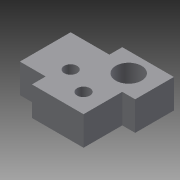
# Autodesk Inventor part: P1-4
Saved by Autodesk Inventor 2014 (Build 180170000, 170)
## iProperties
Created: 2017-02-06
Part Number: P1-4
Material: Generic
Document SubType Name: Modeling
Designer: mschaffel
Density: 1 g/cm^3
Appearance: Default
Author: mschaffel
Autodesk Inventor part; units mm, degrees
ref_plane "YZ Plane" through (0, 0, 0) normal (1, 0, 0) x (0, 1, 0)
ref_plane "XZ Plane" through (0, 0, 0) normal (0, 1, 0) x (-1, 0, 0)
ref_plane "XY Plane" through (0, 0, 0) normal (0, 0, 1) x (1, 0, 0)
sketch "Sketch1" plane through (0, 0, 0) normal (0, 1, 0) x (-1, 0, 0)
  line L0 (0, 0) -> (0, 38.1)
  line L1 (0, 38.1) -> (12.7, 38.1)
  line L2 (12.7, 38.1) -> (12.7, 76.2)
  line L3 (0, 0) -> (50.8, 0)
  line L4 (50.8, 0) -> (50.8, 12.7)
  line L5 (50.8, 12.7) -> (88.9, 12.7)
  line L6 (88.9, 12.7) -> (88.9, 62.673)
  circle A0 centre (25.4, 19.05) radius 12.7
  circle A1 centre (31.75, 57.15) radius 6.35
  line L7 (12.7, 76.2) -> (63.5, 76.2)
  line L8 (63.5, 76.2) -> (63.5, 62.673)
  line L9 (63.5, 62.673) -> (88.9, 62.673)
  circle A2 centre (57.15, 44.45) radius 6.35
  dimension "d0" = 38.1
  dimension "d1" = 50.8
  dimension "d2" = 25.4
  dimension "d3" = 12.7
  dimension "d4" = 12.7
  constraints: 20 end point, 3 centre point, 3 parallel, 2 perpendicular, 1 vertical
  measures "d0" distance of L0.start L0.end
  measures "d1" distance of L0.start L3.end
  measures "d2" diameter of A0
  measures "d3" diameter of A1
  measures "d4" diameter of A2
extrude "Extrusion1" add sketch "Sketch1" along normal blind 28.575
body "Solid1"
